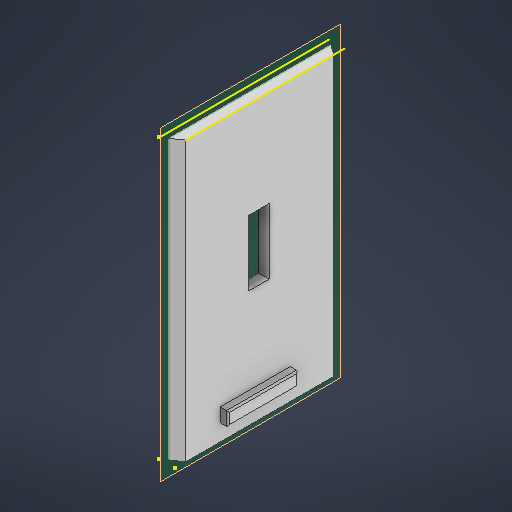
# Autodesk Inventor part: Part2
Saved by Autodesk Inventor 2026.1 (Build 301233000, 233)
## iProperties
Created: 2025-08-25
Part Number: Part2
Material: Generic
Document SubType Name: Modeling
Designer: usman
Density: 1 g/cm^3
Appearance: Default
Author: usman
Autodesk Inventor part; units mm, degrees
(part 1 of 2)
ref_plane "YZ Plane" through (0, 0, 0) normal (1, 0, 0) x (0, 1, 0)
ref_plane "XZ Plane" through (0, 0, 0) normal (0, 1, 0) x (-1, 0, 0)
ref_plane "XY Plane" through (0, 0, 0) normal (0, 0, 1) x (1, 0, 0)
sketch "Sketch1" plane through (0, 0, 0) normal (1, 0, 0) x (0, 1, 0)
  line L0 (0, 0) -> (178.9, 0)
  line L1 (178.9, 0) -> (178.9, -109)
  line L2 (178.9, -109) -> (0, -109)
  line L3 (0, -109) -> (0, 0)
  dimension "d0" = 178.9
  dimension "d1" = 109
  constraints: 8 end point, 2 parallel, 1 horizontal, 1 perpendicular
  measures "d0" distance of L1.end L2.end
  measures "d1" distance of L0.end L1.end
extrude "Extrusion1" add sketch "Sketch1" along normal blind 10
sketch "Sketch2" plane through (0, 178.9, 0) normal (0, 1, 0) x (1, 0, 0)
  point P0 (0, 0)
sketch "Sketch3" plane through (0, 178.9, 0) normal (0, 1, 0) x (1, 0, 0)
  line L0 (0, 109) -> (10, 101.9979)
  line L1 (10, 109) -> (10, 0) projected
  line L2 (0, 109) -> (0, 0) projected
  line L3 (0, 0) -> (10, 0) projected
  line L4 (0, 0) -> (10, 7.0021)
  dimension "d4" = 125
  dimension "d5" = 125
  constraints: 4 end point, 2 point on line
  measures "d4" angle of L2 L0
  measures "d5" angle of L2 L4
extrude "Extrusion2" cut sketch "Sketch3" against normal through all contours L4 L1 L3
sketch "Sketch4" plane through (0, 178.9, -109) normal (0, 1, 0) x (1, 0, 0)
  point P0 (0, -109)
sketch "Sketch5" plane through (0, 178.9, -109) normal (0, 1, 0) x (1, 0, 0)
  line L0 (0, -109) -> (0, 0) projected
  line L1 (10, 0) -> (10, -101.9979) projected
sketch "Sketch6" plane through (0, 178.9, -109) normal (0, 1, 0) x (1, 0, 0)
  line L0 (0, -109) -> (0, 0) projected
  line L1 (0, 0) -> (10, -7.0021)
  line L2 (10, 0) -> (10, -101.9979) projected
  line L3 (0, 0) -> (10, 0)
  line L4 (0, 0) -> (10, 0) projected
  line L5 (10, 0) -> (10, -7.0021)
  dimension "d8" = 125
  constraints: 6 end point, 1 collinear, 1 perpendicular, 1 point on line
  measures "d8" angle of L2 L1
extrude "Extrusion3" cut sketch "Sketch6" against normal through all
sketch "Sketch7" plane through (10, 0, 0) normal (1, 0, 0) x (0, 0, -1)
  point P0 (0, 0)
sketch "Sketch8" plane through (10, 0, 0) normal (1, 0, 0) x (0, 0, -1)
  line L0 (47.4589, 116.9) -> (60.4589, 116.9)
  line L1 (60.4589, 116.9) -> (60.4589, 74.9)
  line L2 (60.4589, 74.9) -> (47.4589, 74.9)
  line L3 (47.4589, 74.9) -> (47.4589, 116.9)
  line L4 (101.9979, 178.9) -> (7.0021, 178.9) projected
  point P0 (0, 0)
  dimension "d11" = 13
  dimension "d12" = 42
  dimension "d13" = 62
  constraints: 8 end point, 2 parallel, 1 horizontal, 1 perpendicular
  measures "d11" distance of L0.start L0.end
  measures "d12" distance of L0.end L1.end
  measures "d13" distance between parallel lines of L0 L4
extrude "Extrusion4" cut sketch "Sketch8" against normal through all
sketch "Sketch9" plane through (0, 0, 0) normal (0.5735764, 0, 0.819152) x (0.819152, 0, -0.5735764)
  point P0 (0, 0)
sketch "Sketch10" plane through (0, 0, 0) normal (0.5735764, 0, 0.819152) x (0.819152, 0, -0.5735764)
  point P0 (0, 0)
sketch "Sketch11" plane through (0, 178.9, 0) normal (0, 1, 0) x (1, 0, 0)
  line L0 (0, 109) -> (0, 0) projected
  line L1 (0, 109) -> (0.5, 109)
  line L2 (0.5, 109) -> (0.5, 0)
  line L3 (0.5, 0) -> (0, 0)
  line L4 (0, 0) -> (0, 109)
  dimension "d16" = 0.5
  constraints: 8 end point, 2 parallel, 1 horizontal, 1 perpendicular
  measures "d16" distance of L2.end L3.end
extrude "Extrusion5" cut sketch "Sketch11" against normal through all
sketch "Sketch12" plane through (10, 0, 0) normal (1, 0, 0) x (0, 0, -1)
  line L0 (73.9981, 10.7247) -> (29.0021, 10.7247)
  line L1 (29.0021, 10.7247) -> (29.0021, 19.4458)
  line L2 (29.0021, 19.4458) -> (73.9981, 19.4458)
  line L3 (73.9981, 19.4458) -> (73.9981, 10.7247)
  line L4 (7.0021, 178.9) -> (7.0021, 0) projected
  point P0 (0, 0)
  point P1 (29.0021, 15.0853)
  dimension "d19" = 22
  dimension "d20" = 44.996
  constraints: 8 end point, 2 parallel, 1 horizontal, 1 midpoint, 1 perpendicular
  measures "d19" distance from line of L4 point (29.002, 15.085)
  measures "d20" distance of L0.start L0.end
extrude "Extrusion6" add sketch "Sketch12" along normal blind 5
fillet "Fillet1" radius 1 4 edges at (15, 19.4458, -51.5001) (15, 10.7247, -51.5001) (15, 15.0853, -29.0021) (15, 15.0853, -73.9981)
sketch "Sketch14" plane through (10, 178.9, -7.0021) normal (0, 1, 0) x (1, 0, 0)
  line L0 (0, 94.9958) -> (-9.5, 101.6478) projected
  line L1 (-9.5, 101.6478) -> (-7, 101.6478)
  line L2 (-7, 101.6478) -> (-7, -6.652)
  line L3 (-7, -6.652) -> (-9.5, -6.652)
  line L4 (-9.5, -6.652) -> (-9.5, 101.6478)
  point P0 (-10, -7.0021)
  dimension "d25" = 2.5
  constraints: 8 end point, 2 parallel, 1 horizontal, 1 perpendicular
  measures "d25" distance of L2.end L3.end
extrude "Extrusion7" cut sketch "Sketch14" against normal through all
ref_plane "Work Plane2" through (4, 178.9, -106.8994) normal (-1, 0, 0) x (0, 0, 1)
sketch "Sketch15" plane through (4, 178.9, -106.8994) normal (-1, 0, 0) x (0, 0, 1)
  arc A0 (103.1758, -166.633) -> (98.1758, -166.633) centre (100.6758, -166.633) ccw
  arc A1 (6.623, -166.633) -> (1.623, -166.633) centre (4.123, -166.633) ccw
  line L0 (104.7988, -178.9) -> (0, -178.9) projected
  line L1 (104.7988, 0) -> (104.7988, -178.9) projected
  line L2 (0, -178.9) -> (0, 0) projected
  line L3 (103.1758, -166.633) -> (98.1758, -166.633)
  line L4 (6.623, -166.633) -> (1.623, -166.633)
  point P0 (106.8994, -178.9)
  dimension "d29" = 12.267
  dimension "d30" = 12.267
  dimension "d31" = 4.123
  dimension "d32" = 4.123
  dimension "d33" = 5
  dimension "d34" = 5
  constraints: 4 end point, 4 point on circle, 2 centre point, 2 point on line, 1 horizontal
  measures "d29" distance from line of A0.centre L0
  measures "d30" distance from line of A1.centre L0
  measures "d31" distance from line of A0.centre L1
  measures "d32" distance from line of L2 A1.centre
  measures "d33" diameter of A0
  measures "d34" diameter of A1
revolve "Revolution1" add sketch "Sketch15" angle 360 about axis through (4, 12.267, -3.7236) along (0, 0, -1)
sketch "Sketch18" plane through (3, 178.9, -106.8994) normal (-1, 0, 0) x (0, 0, 1)
  line L0 (10.7042, -119.5303) -> (95.1976, -119.5303) construction
  line L1 (95.1976, -119.5303) -> (95.1976, -169.3697) construction
  line L2 (95.1976, -169.3697) -> (10.7042, -169.3697) construction
  line L3 (10.7042, -169.3697) -> (10.7042, -119.5303) construction
  line L4 (38.2413, -134.9776) -> (35.8706, -134.9776)
  line L5 (35.8706, -134.9776) -> (35.4573, -135.9339)
  spline S0 degree 2 poles (35.4573, -135.9339) (35.3029, -136.2925) (35.3029, -136.4668) knots 0 0 0 1 1 1
  spline S1 degree 2 poles (35.3029, -136.4668) (35.3029, -136.6062) (35.5718, -136.8204) (36.0101, -136.8503) knots 0 0 0 1 2 2 2
  line L6 (36.0101, -136.8503) -> (36.0101, -137.0146)
  line L7 (36.0101, -137.0146) -> (34.0877, -137.0146)
  line L8 (34.0877, -137.0146) -> (34.0877, -136.8503)
  spline S2 degree 2 poles (34.0877, -136.8503) (34.4711, -136.7805) (34.5807, -136.6759) knots 0 0 0 1 1 1
  spline S3 degree 2 poles (34.5807, -136.6759) (34.8098, -136.4568) (35.0887, -135.7944) knots 0 0 0 1 1 1
  line L9 (35.0887, -135.7944) -> (37.2402, -130.7792)
  line L10 (37.2402, -130.7792) -> (37.3996, -130.7792)
  line L11 (37.3996, -130.7792) -> (39.5213, -135.8492)
  spline S4 degree 2 poles (39.5213, -135.8492) (39.7753, -136.4618) (40.1936, -136.8254) (40.5671, -136.8503) knots 0 0 0 1 2 2 2
  line L12 (40.5671, -136.8503) -> (40.5671, -137.0146)
  line L13 (40.5671, -137.0146) -> (38.1616, -137.0146)
  line L14 (38.1616, -137.0146) -> (38.1616, -136.8503)
  spline S5 degree 2 poles (38.1616, -136.8503) (38.5252, -136.8303) (38.7842, -136.6261) (38.7842, -136.4767) knots 0 0 0 1 2 2 2
  spline S6 degree 2 poles (38.7842, -136.4767) (38.7842, -136.2775) (38.6049, -135.8492) knots 0 0 0 1 1 1
  line L15 (38.6049, -135.8492) -> (38.2413, -134.9776)
  line L16 (38.1019, -134.6439) -> (37.0759, -132.1786)
  line L17 (37.0759, -132.1786) -> (36.0101, -134.6439)
  line L18 (36.0101, -134.6439) -> (38.1019, -134.6439)
  line L19 (44.666, -130.9186) -> (44.3174, -131.6806)
  line L20 (44.3174, -131.6806) -> (42.4846, -131.6806)
  line L21 (42.4846, -131.6806) -> (42.0812, -132.4974)
  spline S7 degree 2 poles (42.0812, -132.4974) (43.2715, -132.6717) (43.9688, -133.3839) knots 0 0 0 1 1 1
  spline S8 degree 2 poles (43.9688, -133.3839) (44.5664, -133.9965) (44.5664, -134.8232) knots 0 0 0 1 1 1
  spline S9 degree 2 poles (44.5664, -134.8232) (44.5664, -135.3014) (44.173, -136.1231) (43.5803, -136.6959) (43.2167, -136.8702) knots 0 0 0 1 2 3 3 3
  spline S10 degree 2 poles (43.2167, -136.8702) (42.6988, -137.1192) (42.1559, -137.1192) knots 0 0 0 1 1 1
  spline S11 degree 2 poles (42.1559, -137.1192) (41.6031, -137.1192) (41.105, -136.7457) (41.105, -136.5216) knots 0 0 0 1 2 2 2
  spline S12 degree 2 poles (41.105, -136.5216) (41.105, -136.397) (41.3092, -136.2028) (41.4686, -136.2028) knots 0 0 0 1 2 2 2
  spline S13 degree 2 poles (41.4686, -136.2028) (41.5831, -136.2028) (41.7624, -136.2775) (41.9716, -136.4269) knots 0 0 0 1 2 2 2
  spline S14 degree 2 poles (41.9716, -136.4269) (42.3103, -136.656) (42.6589, -136.661) knots 0 0 0 1 1 1
  spline S15 degree 2 poles (42.6589, -136.661) (43.1819, -136.661) (43.9837, -135.8641) (43.9837, -135.2914) knots 0 0 0 1 2 2 2
  spline S16 degree 2 poles (43.9837, -135.2914) (43.9837, -134.7386) (43.2715, -133.7774) (42.644, -133.5184) knots 0 0 0 1 2 2 2
  spline S17 degree 2 poles (42.644, -133.5184) (42.1559, -133.3142) (41.3092, -133.2843) knots 0 0 0 1 1 1
  line L22 (41.3092, -133.2843) -> (42.4796, -130.9186)
  line L23 (42.4796, -130.9186) -> (44.666, -130.9186)
  spline S18 degree 2 poles (45.6073, -134.0015) (45.6073, -132.9606) (46.2348, -131.4565) (46.7578, -131.0879) knots 0 0 0 1 2 2 2
  spline S19 degree 2 poles (46.7578, -131.0879) (47.1612, -130.7941) (47.5945, -130.7941) knots 0 0 0 1 1 1
  spline S20 degree 2 poles (47.5945, -130.7941) (48.2967, -130.7941) (48.8545, -131.5063) knots 0 0 0 1 1 1
  spline S21 degree 2 poles (48.8545, -131.5063) (49.5518, -132.3928) (49.5518, -133.9068) knots 0 0 0 1 1 1
  spline S22 degree 2 poles (49.5518, -133.9068) (49.5518, -134.9677) (48.9392, -136.4518) (47.9929, -137.1192) (47.5497, -137.1192) knots 0 0 0 1 2 3 3 3
  spline S23 degree 2 poles (47.5497, -137.1192) (46.6781, -137.1192) (46.0954, -136.0883) knots 0 0 0 1 1 1
  spline S24 degree 2 poles (46.0954, -136.0883) (45.6073, -135.2217) (45.6073, -134.0015) knots 0 0 0 1 1 1
  spline S25 degree 2 poles (46.4888, -134.116) (46.4888, -135.3711) (46.7976, -136.1679) knots 0 0 0 1 1 1
  spline S26 degree 2 poles (46.7976, -136.1679) (47.0566, -136.8353) (47.5646, -136.8353) knots 0 0 0 1 1 1
  spline S27 degree 2 poles (47.5646, -136.8353) (47.8086, -136.8353) (48.3266, -136.402) (48.4611, -135.889) knots 0 0 0 1 2 2 2
  spline S28 degree 2 poles (48.4611, -135.889) (48.6702, -135.1171) (48.6702, -133.7126) knots 0 0 0 1 1 1
  spline S29 degree 2 poles (48.6702, -133.7126) (48.6702, -132.6667) (48.4561, -131.9745) knots 0 0 0 1 1 1
  spline S30 degree 2 poles (48.4561, -131.9745) (48.2917, -131.4565) (48.0377, -131.2423) knots 0 0 0 1 1 1
  spline S31 degree 2 poles (48.0377, -131.2423) (47.8535, -131.0929) (47.5895, -131.0929) knots 0 0 0 1 1 1
  spline S32 degree 2 poles (47.5895, -131.0929) (47.2857, -131.0929) (47.0466, -131.3668) knots 0 0 0 1 1 1
  spline S33 degree 2 poles (47.0466, -131.3668) (46.7229, -131.7404) (46.4888, -133.3391) (46.4888, -134.116) knots 0 0 0 1 2 2 2
  spline S34 degree 2 poles (50.2142, -134.0015) (50.2142, -132.9606) (50.8417, -131.4565) (51.3646, -131.0879) knots 0 0 0 1 2 2 2
  spline S35 degree 2 poles (51.3646, -131.0879) (51.7681, -130.7941) (52.2013, -130.7941) knots 0 0 0 1 1 1
  spline S36 degree 2 poles (52.2013, -130.7941) (52.9036, -130.7941) (53.4614, -131.5063) knots 0 0 0 1 1 1
  spline S37 degree 2 poles (53.4614, -131.5063) (54.1586, -132.3928) (54.1586, -133.9068) knots 0 0 0 1 1 1
  spline S38 degree 2 poles (54.1586, -133.9068) (54.1586, -134.9677) (53.5461, -136.4518) (52.5998, -137.1192) (52.1565, -137.1192) knots 0 0 0 1 2 3 3 3
  spline S39 degree 2 poles (52.1565, -137.1192) (51.285, -137.1192) (50.7022, -136.0883) knots 0 0 0 1 1 1
  spline S40 degree 2 poles (50.7022, -136.0883) (50.2142, -135.2217) (50.2142, -134.0015) knots 0 0 0 1 1 1
  spline S41 degree 2 poles (51.0957, -134.116) (51.0957, -135.3711) (51.4045, -136.1679) knots 0 0 0 1 1 1
  spline S42 degree 2 poles (51.4045, -136.1679) (51.6635, -136.8353) (52.1715, -136.8353) knots 0 0 0 1 1 1
  spline S43 degree 2 poles (52.1715, -136.8353) (52.4155, -136.8353) (52.9335, -136.402) (53.0679, -135.889) knots 0 0 0 1 2 2 2
  spline S44 degree 2 poles (53.0679, -135.889) (53.2771, -135.1171) (53.2771, -133.7126) knots 0 0 0 1 1 1
  spline S45 degree 2 poles (53.2771, -133.7126) (53.2771, -132.6667) (53.063, -131.9745) knots 0 0 0 1 1 1
  spline S46 degree 2 poles (53.063, -131.9745) (52.8986, -131.4565) (52.6446, -131.2423) knots 0 0 0 1 1 1
  spline S47 degree 2 poles (52.6446, -131.2423) (52.4603, -131.0929) (52.1964, -131.0929) knots 0 0 0 1 1 1
  spline S48 degree 2 poles (52.1964, -131.0929) (51.8926, -131.0929) (51.6535, -131.3668) knots 0 0 0 1 1 1
  spline S49 degree 2 poles (51.6535, -131.3668) (51.3298, -131.7404) (51.0957, -133.3391) (51.0957, -134.116) knots 0 0 0 1 2 2 2
  line L24 (59.1739, -138.9968) -> (54.4126, -138.9968)
  line L25 (54.4126, -138.9968) -> (54.4126, -138.6183)
  line L26 (54.4126, -138.6183) -> (59.1739, -138.6183)
  line L27 (59.1739, -138.6183) -> (59.1739, -138.9968)
  line L28 (64.3734, -135.3263) -> (64.5228, -135.3561)
  line L29 (64.5228, -135.3561) -> (63.9999, -137.0146)
  line L30 (63.9999, -137.0146) -> (59.2835, -137.0146)
  line L31 (59.2835, -137.0146) -> (59.2835, -136.8503)
  line L32 (59.2835, -136.8503) -> (59.5126, -136.8503)
  spline S50 degree 2 poles (59.5126, -136.8503) (59.8961, -136.8503) (60.0604, -136.5963) knots 0 0 0 1 1 1
  spline S51 degree 2 poles (60.0604, -136.5963) (60.155, -136.4568) (60.155, -135.9339) knots 0 0 0 1 1 1
  line L33 (60.155, -135.9339) -> (60.155, -131.9994)
  spline S52 degree 2 poles (60.155, -131.9994) (60.155, -131.4266) (60.0305, -131.2822) knots 0 0 0 1 1 1
  spline S53 degree 2 poles (60.0305, -131.2822) (59.8562, -131.083) (59.5126, -131.083) knots 0 0 0 1 1 1
  line L34 (59.5126, -131.083) -> (59.2835, -131.083)
  line L35 (59.2835, -131.083) -> (59.2835, -130.9186)
  line L36 (59.2835, -130.9186) -> (62.0376, -130.9186)
  line L37 (62.0376, -130.9186) -> (62.0376, -131.083)
  spline S54 degree 2 poles (62.0376, -131.083) (61.5495, -131.078) (61.1611, -131.2672) (61.0166, -131.5561) (61.0166, -132.099) knots 0 0 0 1 2 3 3 3
  line L38 (61.0166, -132.099) -> (61.0166, -135.9289)
  spline S55 degree 2 poles (61.0166, -135.9289) (61.0166, -136.3024) (61.0864, -136.4419) knots 0 0 0 1 1 1
  spline S56 degree 2 poles (61.0864, -136.4419) (61.1411, -136.5365) (61.3653, -136.6261) (61.9579, -136.6261) knots 0 0 0 1 2 2 2
  line L39 (61.9579, -136.6261) -> (62.4012, -136.6261)
  spline S57 degree 2 poles (62.4012, -136.6261) (63.1034, -136.6261) (63.6712, -136.417) (64.1393, -135.894) (64.3734, -135.3263) knots 0 0 0 1 2 3 3 3
  line L40 (66.4253, -132.7763) -> (66.4253, -136.0833)
  spline S58 degree 2 poles (66.4253, -136.0833) (66.4253, -136.4668) (66.5349, -136.7257) (66.759, -136.8503) (67.0479, -136.8503) knots 0 0 0 1 2 3 3 3
  line L41 (67.0479, -136.8503) -> (67.0479, -137.0146)
  line L42 (67.0479, -137.0146) -> (65.0508, -137.0146)
  line L43 (65.0508, -137.0146) -> (65.0508, -136.8503)
  spline S59 degree 2 poles (65.0508, -136.8503) (65.3496, -136.8503) (65.5588, -136.7357) (65.6783, -136.4668) (65.6783, -136.0833) knots 0 0 0 1 2 3 3 3
  line L44 (65.6783, -136.0833) -> (65.6783, -134.4995)
  spline S60 degree 2 poles (65.6783, -134.4995) (65.6783, -133.8321) (65.6384, -133.6329) knots 0 0 0 1 1 1
  spline S61 degree 2 poles (65.6384, -133.6329) (65.6086, -133.4885) (65.4691, -133.3739) (65.3546, -133.3739) knots 0 0 0 1 2 2 2
  spline S62 degree 2 poles (65.3546, -133.3739) (65.2301, -133.3739) (65.0508, -133.4437) knots 0 0 0 1 1 1
  line L45 (65.0508, -133.4437) -> (64.986, -133.2793)
  line L46 (64.986, -133.2793) -> (66.2261, -132.7763)
  line L47 (66.2261, -132.7763) -> (66.4253, -132.7763)
  spline S63 degree 2 poles (66.0518, -130.6198) (66.2411, -130.6198) (66.505, -130.8837) (66.505, -131.073) knots 0 0 0 1 2 2 2
  spline S64 degree 2 poles (66.505, -131.073) (66.505, -131.2623) (66.2411, -131.5312) (66.0518, -131.5312) knots 0 0 0 1 2 2 2
  spline S65 degree 2 poles (66.0518, -131.5312) (65.8626, -131.5312) (65.5936, -131.2623) (65.5936, -131.073) knots 0 0 0 1 2 2 2
  spline S66 degree 2 poles (65.5936, -131.073) (65.5936, -130.8837) (65.8576, -130.6198) (66.0518, -130.6198) knots 0 0 0 1 2 2 2
  spline S67 degree 2 poles (70.4694, -136.5514) (70.1706, -136.8652) (69.5929, -137.1391) (69.2592, -137.1391) knots 0 0 0 1 2 2 2
  spline S68 degree 2 poles (69.2592, -137.1391) (68.5868, -137.1391) (67.5808, -136.0136) (67.5808, -135.127) knots 0 0 0 1 2 2 2
  spline S69 degree 2 poles (67.5808, -135.127) (67.5808, -134.2455) (68.6964, -132.7763) (69.573, -132.7763) knots 0 0 0 1 2 2 2
  spline S70 degree 2 poles (69.573, -132.7763) (70.1158, -132.7763) (70.4694, -133.1249) knots 0 0 0 1 1 1
  line L48 (70.4694, -133.1249) -> (70.4694, -132.353)
  spline S71 degree 2 poles (70.4694, -132.353) (70.4694, -131.6507) (70.3997, -131.332) (70.2602, -131.2174) (70.1507, -131.2174) knots 0 0 0 1 2 3 3 3
  spline S72 degree 2 poles (70.1507, -131.2174) (70.0361, -131.2174) (69.8419, -131.2872) knots 0 0 0 1 1 1
  line L49 (69.8419, -131.2872) -> (69.7821, -131.1228)
  line L50 (69.7821, -131.1228) -> (71.0073, -130.6198)
  line L51 (71.0073, -130.6198) -> (71.2115, -130.6198)
  line L52 (71.2115, -130.6198) -> (71.2115, -135.386)
  spline S73 degree 2 poles (71.2115, -135.386) (71.2115, -136.1032) (71.2812, -136.4219) (71.4257, -136.5465) (71.5253, -136.5465) knots 0 0 0 1 2 3 3 3
  spline S74 degree 2 poles (71.5253, -136.5465) (71.6448, -136.5465) (71.849, -136.4717) knots 0 0 0 1 1 1
  line L53 (71.849, -136.4717) -> (71.8988, -136.6361)
  line L54 (71.8988, -136.6361) -> (70.6786, -137.1391)
  line L55 (70.6786, -137.1391) -> (70.4694, -137.1391)
  line L56 (70.4694, -137.1391) -> (70.4694, -136.5514)
  line L57 (70.4694, -136.2327) -> (70.4694, -134.121)
  spline S75 degree 2 poles (70.4694, -134.121) (70.4445, -133.8122) (70.1706, -133.3092) (69.7273, -133.0552) (69.5182, -133.0552) knots 0 0 0 1 2 3 3 3
  spline S76 degree 2 poles (69.5182, -133.0552) (69.1197, -133.0552) (68.811, -133.4088) knots 0 0 0 1 1 1
  spline S77 degree 2 poles (68.811, -133.4088) (68.4026, -133.877) (68.4026, -134.7734) knots 0 0 0 1 1 1
  spline S78 degree 2 poles (68.4026, -134.7734) (68.4026, -135.6799) (69.1944, -136.6461) (69.6775, -136.6461) knots 0 0 0 1 2 2 2
  spline S79 degree 2 poles (69.6775, -136.6461) (70.0859, -136.6461) (70.4694, -136.2327) knots 0 0 0 1 1 1
  line L58 (17.7843, -140.4209) -> (17.7843, -142.5276)
  line L59 (17.7843, -142.5276) -> (17.62, -142.5276)
  spline S80 degree 2 poles (17.62, -142.5276) (17.5403, -141.9199) (17.117, -141.2028) (16.345, -140.7794) (15.9267, -140.7794) knots 0 0 0 1 2 3 3 3
  spline S81 degree 2 poles (15.9267, -140.7794) (15.4585, -140.7794) (14.8459, -141.3522) (14.8459, -141.7158) knots 0 0 0 1 2 2 2
  spline S82 degree 2 poles (14.8459, -141.7158) (14.8459, -141.9947) (15.0401, -142.2238) knots 0 0 0 1 1 1
  spline S83 degree 2 poles (15.0401, -142.2238) (15.319, -142.5624) (16.3699, -143.1252) knots 0 0 0 1 1 1
  spline S84 degree 2 poles (16.3699, -143.1252) (17.2216, -143.5834) (17.8491, -144.0715) (18.1878, -144.7389) (18.1878, -145.1024) knots 0 0 0 1 2 3 3 3
  spline S85 degree 2 poles (18.1878, -145.1024) (18.1878, -145.7947) (17.112, -146.7958) (16.2653, -146.7958) knots 0 0 0 1 2 2 2
  spline S86 degree 2 poles (16.2653, -146.7958) (16.0014, -146.7958) (15.7673, -146.7559) knots 0 0 0 1 1 1
  spline S87 degree 2 poles (15.7673, -146.7559) (15.6278, -146.731) (14.7513, -146.4471) (14.6318, -146.4471) knots 0 0 0 1 2 2 2
  spline S88 degree 2 poles (14.6318, -146.4471) (14.5222, -146.4471) (14.3877, -146.5816) (14.3578, -146.7958) knots 0 0 0 1 2 2 2
  line L60 (14.3578, -146.7958) -> (14.1935, -146.7958)
  line L61 (14.1935, -146.7958) -> (14.1935, -144.704)
  line L62 (14.1935, -144.704) -> (14.3578, -144.704)
  spline S89 degree 2 poles (14.3578, -144.704) (14.4724, -145.3614) (14.8708, -146.0138) (15.6876, -146.4471) (16.1707, -146.4471) knots 0 0 0 1 2 3 3 3
  spline S90 degree 2 poles (16.1707, -146.4471) (16.7335, -146.4471) (17.3859, -145.8545) (17.3859, -145.4461) knots 0 0 0 1 2 2 2
  spline S91 degree 2 poles (17.3859, -145.4461) (17.3859, -145.2219) (17.1369, -144.7638) (16.8779, -144.5645) knots 0 0 0 1 2 2 2
  spline S92 degree 2 poles (16.8779, -144.5645) (16.7036, -144.4301) (15.1348, -143.5535) (14.4724, -143.0306) (14.1287, -142.403) (14.1287, -142.0245) knots 0 0 0 1 2 3 4 4 4
  spline S93 degree 2 poles (14.1287, -142.0245) (14.1287, -141.3671) (15.1398, -140.4209) (15.9217, -140.4209) knots 0 0 0 1 2 2 2
  spline S94 degree 2 poles (15.9217, -140.4209) (16.4048, -140.4209) (16.9526, -140.6599) knots 0 0 0 1 1 1
  spline S95 degree 2 poles (16.9526, -140.6599) (17.2066, -140.7695) (17.3112, -140.7695) knots 0 0 0 1 1 1
  spline S96 degree 2 poles (17.3112, -140.7695) (17.4258, -140.7695) (17.5752, -140.63) (17.62, -140.4209) knots 0 0 0 1 2 2 2
  line L63 (17.62, -140.4209) -> (17.7843, -140.4209)
  spline S97 degree 2 poles (19.652, -144.0914) (19.647, -145.0078) (20.0952, -145.5258) knots 0 0 0 1 1 1
  spline S98 degree 2 poles (20.0952, -145.5258) (20.5485, -146.0487) (21.1561, -146.0487) knots 0 0 0 1 1 1
  spline S99 degree 2 poles (21.1561, -146.0487) (21.5595, -146.0487) (22.1571, -145.6054) (22.3613, -145.0626) knots 0 0 0 1 2 2 2
  line L64 (22.3613, -145.0626) -> (22.5008, -145.1522)
  spline S100 degree 2 poles (22.5008, -145.1522) (22.4061, -145.7698) (21.4997, -146.7808) (20.8124, -146.7808) knots 0 0 0 1 2 2 2
  spline S101 degree 2 poles (20.8124, -146.7808) (20.0703, -146.7808) (19.0145, -145.6254) (19.0145, -144.6542) knots 0 0 0 1 2 2 2
  spline S102 degree 2 poles (19.0145, -144.6542) (19.0145, -143.5983) (20.1002, -142.418) (20.917, -142.418) knots 0 0 0 1 2 2 2
  spline S103 degree 2 poles (20.917, -142.418) (21.6093, -142.418) (22.5008, -143.3294) (22.5008, -144.0914) knots 0 0 0 1 2 2 2
  line L65 (22.5008, -144.0914) -> (19.652, -144.0914)
  line L66 (19.652, -143.8324) -> (21.5645, -143.8324)
  spline S104 degree 2 poles (21.5645, -143.8324) (21.5396, -143.439) (21.4698, -143.2746) knots 0 0 0 1 1 1
  spline S105 degree 2 poles (21.4698, -143.2746) (21.3553, -143.0256) (20.912, -142.7367) (20.668, -142.7367) knots 0 0 0 1 2 2 2
  spline S106 degree 2 poles (20.668, -142.7367) (20.2945, -142.7367) (19.7018, -143.3145) (19.652, -143.8324) knots 0 0 0 1 2 2 2
  line L67 (24.2589, -142.418) -> (24.2589, -143.3443)
  spline S107 degree 2 poles (24.2589, -143.3443) (24.7768, -142.418) (25.3197, -142.418) knots 0 0 0 1 1 1
  spline S108 degree 2 poles (25.3197, -142.418) (25.5637, -142.418) (25.8874, -142.7168) (25.8874, -142.916) knots 0 0 0 1 2 2 2
  spline S109 degree 2 poles (25.8874, -142.916) (25.8874, -143.0903) (25.6534, -143.3344) (25.494, -143.3344) knots 0 0 0 1 2 2 2
  spline S110 degree 2 poles (25.494, -143.3344) (25.3346, -143.3344) (24.9461, -143.0256) (24.8515, -143.0256) knots 0 0 0 1 2 2 2
  spline S111 degree 2 poles (24.8515, -143.0256) (24.7718, -143.0256) (24.6772, -143.1152) knots 0 0 0 1 1 1
  spline S112 degree 2 poles (24.6772, -143.1152) (24.473, -143.2995) (24.2589, -143.7229) knots 0 0 0 1 1 1
  line L68 (24.2589, -143.7229) -> (24.2589, -145.6951)
  spline S113 degree 2 poles (24.2589, -145.6951) (24.2589, -146.0387) (24.3435, -146.213) knots 0 0 0 1 1 1
  spline S114 degree 2 poles (24.3435, -146.213) (24.4033, -146.3326) (24.6971, -146.4919) (24.976, -146.4919) knots 0 0 0 1 2 2 2
  line L69 (24.976, -146.4919) -> (24.976, -146.6563)
  line L70 (24.976, -146.6563) -> (22.8643, -146.6563)
  line L71 (22.8643, -146.6563) -> (22.8643, -146.4919)
  spline S115 degree 2 poles (22.8643, -146.4919) (23.1781, -146.4919) (23.3325, -146.3923) knots 0 0 0 1 1 1
  spline S116 degree 2 poles (23.3325, -146.3923) (23.4421, -146.3226) (23.4869, -146.1632) knots 0 0 0 1 1 1
  spline S117 degree 2 poles (23.4869, -146.1632) (23.5118, -146.0836) (23.5118, -145.725) knots 0 0 0 1 1 1
  line L72 (23.5118, -145.725) -> (23.5118, -144.1362)
  spline S118 degree 2 poles (23.5118, -144.1362) (23.5118, -143.419) (23.452, -143.1451) (23.2976, -143.0156) (23.1781, -143.0156) knots 0 0 0 1 2 3 3 3
  spline S119 degree 2 poles (23.1781, -143.0156) (23.0387, -143.0156) (22.8643, -143.0854) knots 0 0 0 1 1 1
  line L73 (22.8643, -143.0854) -> (22.8195, -142.921)
  line L74 (22.8195, -142.921) -> (24.0696, -142.418)
  line L75 (24.0696, -142.418) -> (24.2589, -142.418)
  line L76 (27.536, -142.418) -> (27.536, -145.725)
  spline S120 degree 2 poles (27.536, -145.725) (27.536, -146.1085) (27.6455, -146.3674) (27.8696, -146.4919) (28.1585, -146.4919) knots 0 0 0 1 2 3 3 3
  line L77 (28.1585, -146.4919) -> (28.1585, -146.6563)
  line L78 (28.1585, -146.6563) -> (26.1614, -146.6563)
  line L79 (26.1614, -146.6563) -> (26.1614, -146.4919)
  spline S121 degree 2 poles (26.1614, -146.4919) (26.4602, -146.4919) (26.6694, -146.3774) (26.7889, -146.1085) (26.7889, -145.725) knots 0 0 0 1 2 3 3 3
  line L80 (26.7889, -145.725) -> (26.7889, -144.1412)
  spline S122 degree 2 poles (26.7889, -144.1412) (26.7889, -143.4738) (26.749, -143.2746) knots 0 0 0 1 1 1
  spline S123 degree 2 poles (26.749, -143.2746) (26.7192, -143.1302) (26.5797, -143.0156) (26.4652, -143.0156) knots 0 0 0 1 2 2 2
  spline S124 degree 2 poles (26.4652, -143.0156) (26.3407, -143.0156) (26.1614, -143.0854) knots 0 0 0 1 1 1
  line L81 (26.1614, -143.0854) -> (26.0966, -142.921)
  line L82 (26.0966, -142.921) -> (27.3367, -142.418)
  line L83 (27.3367, -142.418) -> (27.536, -142.418)
  spline S125 degree 2 poles (27.1624, -140.2615) (27.3517, -140.2615) (27.6156, -140.5254) (27.6156, -140.7147) knots 0 0 0 1 2 2 2
  spline S126 degree 2 poles (27.6156, -140.7147) (27.6156, -140.9039) (27.3517, -141.1729) (27.1624, -141.1729) knots 0 0 0 1 2 2 2
  spline S127 degree 2 poles (27.1624, -141.1729) (26.9732, -141.1729) (26.7042, -140.9039) (26.7042, -140.7147) knots 0 0 0 1 2 2 2
  spline S128 degree 2 poles (26.7042, -140.7147) (26.7042, -140.5254) (26.9682, -140.2615) (27.1624, -140.2615) knots 0 0 0 1 2 2 2
  spline S129 degree 2 poles (31.0073, -146.0587) (30.3748, -146.5517) (30.2104, -146.6264) knots 0 0 0 1 1 1
  spline S130 degree 2 poles (30.2104, -146.6264) (29.9714, -146.741) (29.6974, -146.741) knots 0 0 0 1 1 1
  spline S131 degree 2 poles (29.6974, -146.741) (29.2691, -146.741) (28.7163, -146.1583) (28.7163, -145.6801) knots 0 0 0 1 2 2 2
  spline S132 degree 2 poles (28.7163, -145.6801) (28.7163, -145.3813) (28.8508, -145.1572) knots 0 0 0 1 1 1
  spline S133 degree 2 poles (28.8508, -145.1572) (29.035, -144.8534) (29.9465, -144.3155) (31.0073, -143.927) knots 0 0 0 1 2 2 2
  line L84 (31.0073, -143.927) -> (31.0073, -143.7677)
  spline S134 degree 2 poles (31.0073, -143.7677) (31.0073, -143.1501) (30.6188, -142.6919) (30.2453, -142.6919) knots 0 0 0 1 2 2 2
  spline S135 degree 2 poles (30.2453, -142.6919) (29.9664, -142.6919) (29.797, -142.8463) knots 0 0 0 1 1 1
  spline S136 degree 2 poles (29.797, -142.8463) (29.6277, -142.9957) (29.6277, -143.1949) knots 0 0 0 1 1 1
  line L85 (29.6277, -143.1949) -> (29.6377, -143.4539)
  spline S137 degree 2 poles (29.6377, -143.4539) (29.6377, -143.6631) (29.4235, -143.8872) (29.2542, -143.8872) knots 0 0 0 1 2 2 2
  spline S138 degree 2 poles (29.2542, -143.8872) (29.0898, -143.8872) (28.8757, -143.6531) (28.8757, -143.4489) knots 0 0 0 1 2 2 2
  spline S139 degree 2 poles (28.8757, -143.4489) (28.8757, -143.0654) (29.6676, -142.418) (30.3798, -142.418) knots 0 0 0 1 2 2 2
  spline S140 degree 2 poles (30.3798, -142.418) (30.9276, -142.418) (31.2762, -142.6023) knots 0 0 0 1 1 1
  spline S141 degree 2 poles (31.2762, -142.6023) (31.5452, -142.7417) (31.6697, -143.0356) knots 0 0 0 1 1 1
  spline S142 degree 2 poles (31.6697, -143.0356) (31.7494, -143.2298) (31.7494, -143.8274) knots 0 0 0 1 1 1
  line L86 (31.7494, -143.8274) -> (31.7494, -145.2269)
  spline S143 degree 2 poles (31.7494, -145.2269) (31.7494, -145.8146) (31.7942, -146.0786) (31.8988, -146.1682) (31.9635, -146.1682) knots 0 0 0 1 2 3 3 3
  spline S144 degree 2 poles (31.9635, -146.1682) (32.0382, -146.1682) (32.093, -146.1383) knots 0 0 0 1 1 1
  spline S145 degree 2 poles (32.093, -146.1383) (32.1876, -146.0786) (32.4566, -145.8096) knots 0 0 0 1 1 1
  line L87 (32.4566, -145.8096) -> (32.4566, -146.0587)
  spline S146 degree 2 poles (32.4566, -146.0587) (31.9536, -146.736) (31.4954, -146.736) knots 0 0 0 1 1 1
  spline S147 degree 2 poles (31.4954, -146.736) (31.2712, -146.736) (31.0123, -146.4322) (31.0073, -146.0587) knots 0 0 0 1 2 2 2
  line L88 (31.0073, -145.7698) -> (31.0073, -144.201)
  spline S148 degree 2 poles (31.0073, -144.201) (30.33, -144.4699) (30.1307, -144.5845) knots 0 0 0 1 1 1
  spline S149 degree 2 poles (30.1307, -144.5845) (29.7771, -144.7787) (29.4733, -145.212) (29.4733, -145.466) knots 0 0 0 1 2 2 2
  spline S150 degree 2 poles (29.4733, -145.466) (29.4733, -145.7897) (29.8568, -146.218) (30.1108, -146.218) knots 0 0 0 1 2 2 2
  spline S151 degree 2 poles (30.1108, -146.218) (30.4495, -146.218) (31.0073, -145.7698) knots 0 0 0 1 1 1
  line L89 (34.1848, -140.2615) -> (34.1848, -145.725)
  spline S152 degree 2 poles (34.1848, -145.725) (34.1848, -146.1085) (34.2993, -146.3625) (34.5334, -146.4919) (34.8521, -146.4919) knots 0 0 0 1 2 3 3 3
  line L90 (34.8521, -146.4919) -> (34.8521, -146.6563)
  line L91 (34.8521, -146.6563) -> (32.8251, -146.6563)
  line L92 (32.8251, -146.6563) -> (32.8251, -146.4919)
  spline S153 degree 2 poles (32.8251, -146.4919) (33.109, -146.4919) (33.3182, -146.3774) (33.4377, -146.1085) (33.4377, -145.725) knots 0 0 0 1 2 3 3 3
  line L93 (33.4377, -145.725) -> (33.4377, -141.9847)
  spline S154 degree 2 poles (33.4377, -141.9847) (33.4377, -141.2924) (33.373, -140.9737) (33.2335, -140.8591) (33.1289, -140.8591) knots 0 0 0 1 2 3 3 3
  spline S155 degree 2 poles (33.1289, -140.8591) (33.0094, -140.8591) (32.8301, -140.9289) knots 0 0 0 1 1 1
  line L94 (32.8301, -140.9289) -> (32.7554, -140.7645)
  line L95 (32.7554, -140.7645) -> (33.9806, -140.2615)
  line L96 (33.9806, -140.2615) -> (34.1848, -140.2615)
  line L97 (37.2178, -140.5603) -> (38.8614, -140.5603)
  line L98 (38.8614, -140.5603) -> (42.5967, -145.1373)
  line L99 (42.5967, -145.1373) -> (42.5967, -141.6161)
  spline S156 degree 2 poles (42.5967, -141.6161) (42.5967, -141.0534) (42.4721, -140.9139) knots 0 0 0 1 1 1
  spline S157 degree 2 poles (42.4721, -140.9139) (42.3028, -140.7247) (41.9442, -140.7247) knots 0 0 0 1 1 1
  line L100 (41.9442, -140.7247) -> (41.735, -140.7247)
  line L101 (41.735, -140.7247) -> (41.735, -140.5603)
  line L102 (41.735, -140.5603) -> (43.8517, -140.5603)
  line L103 (43.8517, -140.5603) -> (43.8517, -140.7247)
  line L104 (43.8517, -140.7247) -> (43.6376, -140.7247)
  spline S158 degree 2 poles (43.6376, -140.7247) (43.2491, -140.7247) (43.0897, -140.9587) knots 0 0 0 1 1 1
  spline S159 degree 2 poles (43.0897, -140.9587) (42.9901, -141.1032) (42.9901, -141.6161) knots 0 0 0 1 1 1
  line L105 (42.9901, -141.6161) -> (42.9901, -146.7559)
  line L106 (42.9901, -146.7559) -> (42.8307, -146.7559)
  line L107 (42.8307, -146.7559) -> (38.8116, -141.8452)
  line L108 (38.8116, -141.8452) -> (38.8116, -145.6005)
  spline S160 degree 2 poles (38.8116, -145.6005) (38.8116, -146.1632) (38.9311, -146.3027) knots 0 0 0 1 1 1
  spline S161 degree 2 poles (38.9311, -146.3027) (39.1054, -146.4919) (39.459, -146.4919) knots 0 0 0 1 1 1
  line L109 (39.459, -146.4919) -> (39.6732, -146.4919)
  line L110 (39.6732, -146.4919) -> (39.6732, -146.6563)
  line L111 (39.6732, -146.6563) -> (37.5565, -146.6563)
  line L112 (37.5565, -146.6563) -> (37.5565, -146.4919)
  line L113 (37.5565, -146.4919) -> (37.7657, -146.4919)
  spline S162 degree 2 poles (37.7657, -146.4919) (38.1591, -146.4919) (38.3185, -146.2579) knots 0 0 0 1 1 1
  spline S163 degree 2 poles (38.3185, -146.2579) (38.4181, -146.1134) (38.4181, -145.6005) knots 0 0 0 1 1 1
  line L114 (38.4181, -145.6005) -> (38.4181, -141.3621)
  spline S164 degree 2 poles (38.4181, -141.3621) (38.1541, -141.0484) (37.8802, -140.8492) (37.6113, -140.7645) knots 0 0 0 1 2 2 2
  spline S165 degree 2 poles (37.6113, -140.7645) (37.4818, -140.7247) (37.2178, -140.7247) knots 0 0 0 1 1 1
  line L115 (37.2178, -140.7247) -> (37.2178, -140.5603)
  spline S166 degree 2 poles (46.2871, -142.418) (47.2234, -142.418) (47.7862, -143.1302) knots 0 0 0 1 1 1
  spline S167 degree 2 poles (47.7862, -143.1302) (48.2693, -143.7328) (48.2693, -144.5197) knots 0 0 0 1 1 1
  spline S168 degree 2 poles (48.2693, -144.5197) (48.2693, -145.0725) (47.7364, -146.2081) (46.8101, -146.7808) (46.2373, -146.7808) knots 0 0 0 1 2 3 3 3
  spline S169 degree 2 poles (46.2373, -146.7808) (45.306, -146.7808) (44.7581, -146.0387) knots 0 0 0 1 1 1
  spline S170 degree 2 poles (44.7581, -146.0387) (44.295, -145.4162) (44.295, -144.6392) knots 0 0 0 1 1 1
  spline S171 degree 2 poles (44.295, -144.6392) (44.295, -144.0715) (44.8578, -142.9509) (45.7741, -142.418) (46.2871, -142.418) knots 0 0 0 1 2 3 3 3
  spline S172 degree 2 poles (46.1477, -142.7118) (45.9086, -142.7118) (45.4305, -142.9957) (45.1317, -143.7029) (45.1317, -144.2607) knots 0 0 0 1 2 3 3 3
  spline S173 degree 2 poles (45.1317, -144.2607) (45.1317, -145.1572) (45.8439, -146.4621) (46.4316, -146.4621) knots 0 0 0 1 2 2 2
  spline S174 degree 2 poles (46.4316, -146.4621) (46.8649, -146.4621) (47.4326, -145.7449) (47.4326, -144.8683) knots 0 0 0 1 2 2 2
  spline S175 degree 2 poles (47.4326, -144.8683) (47.4326, -143.7727) (46.9595, -143.1451) knots 0 0 0 1 1 1
  spline S176 degree 2 poles (46.9595, -143.1451) (46.6407, -142.7118) (46.1477, -142.7118) knots 0 0 0 1 1 1
  spline S177 degree 2 poles (49.883, -145.7847) (50.0921, -145.7847) (50.381, -146.0786) (50.381, -146.2828) knots 0 0 0 1 2 2 2
  spline S178 degree 2 poles (50.381, -146.2828) (50.381, -146.4919) (50.0872, -146.7808) (49.883, -146.7808) knots 0 0 0 1 2 2 2
  spline S179 degree 2 poles (49.883, -146.7808) (49.6738, -146.7808) (49.3849, -146.4919) (49.3849, -146.2828) knots 0 0 0 1 2 2 2
  spline S180 degree 2 poles (49.3849, -146.2828) (49.3849, -146.0786) (49.6738, -145.7847) (49.883, -145.7847) knots 0 0 0 1 2 2 2
  spline S181 degree 2 poles (49.8929, -142.418) (50.0971, -142.418) (50.391, -142.7118) (50.391, -142.916) knots 0 0 0 1 2 2 2
  spline S182 degree 2 poles (50.391, -142.916) (50.391, -143.1202) (50.0971, -143.4141) (49.8929, -143.4141) knots 0 0 0 1 2 2 2
  spline S183 degree 2 poles (49.8929, -143.4141) (49.6887, -143.4141) (49.3949, -143.1202) (49.3949, -142.916) knots 0 0 0 1 2 2 2
  spline S184 degree 2 poles (49.3949, -142.916) (49.3949, -142.7118) (49.6887, -142.418) (49.8929, -142.418) knots 0 0 0 1 2 2 2
  line L116 (57.6773, -144.6193) -> (55.3066, -144.6193)
  line L117 (55.3066, -144.6193) -> (54.8932, -145.5756)
  spline S185 degree 2 poles (54.8932, -145.5756) (54.7389, -145.9341) (54.7389, -146.1085) knots 0 0 0 1 1 1
  spline S186 degree 2 poles (54.7389, -146.1085) (54.7389, -146.2479) (55.0078, -146.4621) (55.4461, -146.4919) knots 0 0 0 1 2 2 2
  line L118 (55.4461, -146.4919) -> (55.4461, -146.6563)
  line L119 (55.4461, -146.6563) -> (53.5236, -146.6563)
  line L120 (53.5236, -146.6563) -> (53.5236, -146.4919)
  spline S187 degree 2 poles (53.5236, -146.4919) (53.9071, -146.4222) (54.0167, -146.3176) knots 0 0 0 1 1 1
  spline S188 degree 2 poles (54.0167, -146.3176) (54.2458, -146.0985) (54.5247, -145.4361) knots 0 0 0 1 1 1
  line L121 (54.5247, -145.4361) -> (56.6762, -140.4209)
  line L122 (56.6762, -140.4209) -> (56.8356, -140.4209)
  line L123 (56.8356, -140.4209) -> (58.9572, -145.4909)
  spline S189 degree 2 poles (58.9572, -145.4909) (59.2112, -146.1035) (59.6296, -146.467) (60.0031, -146.4919) knots 0 0 0 1 2 2 2
  line L124 (60.0031, -146.4919) -> (60.0031, -146.6563)
  line L125 (60.0031, -146.6563) -> (57.5976, -146.6563)
  line L126 (57.5976, -146.6563) -> (57.5976, -146.4919)
  spline S190 degree 2 poles (57.5976, -146.4919) (57.9612, -146.472) (58.2201, -146.2678) (58.2201, -146.1184) knots 0 0 0 1 2 2 2
  spline S191 degree 2 poles (58.2201, -146.1184) (58.2201, -145.9192) (58.0409, -145.4909) knots 0 0 0 1 1 1
  line L127 (58.0409, -145.4909) -> (57.6773, -144.6193)
  line L128 (57.5378, -144.2856) -> (56.5119, -141.8203)
  line L129 (56.5119, -141.8203) -> (55.4461, -144.2856)
  line L130 (55.4461, -144.2856) -> (57.5378, -144.2856)
  spline S192 degree 2 poles (60.4364, -143.6432) (60.4364, -142.6023) (61.064, -141.0982) (61.5869, -140.7296) knots 0 0 0 1 2 2 2
  spline S193 degree 2 poles (61.5869, -140.7296) (61.9903, -140.4358) (62.4236, -140.4358) knots 0 0 0 1 1 1
  spline S194 degree 2 poles (62.4236, -140.4358) (63.1258, -140.4358) (63.6836, -141.148) knots 0 0 0 1 1 1
  spline S195 degree 2 poles (63.6836, -141.148) (64.3809, -142.0345) (64.3809, -143.5485) knots 0 0 0 1 1 1
  spline S196 degree 2 poles (64.3809, -143.5485) (64.3809, -144.6094) (63.7683, -146.0935) (62.822, -146.7609) (62.3788, -146.7609) knots 0 0 0 1 2 3 3 3
  spline S197 degree 2 poles (62.3788, -146.7609) (61.5072, -146.7609) (60.9245, -145.7299) knots 0 0 0 1 1 1
  spline S198 degree 2 poles (60.9245, -145.7299) (60.4364, -144.8634) (60.4364, -143.6432) knots 0 0 0 1 1 1
  spline S199 degree 2 poles (61.318, -143.7577) (61.318, -145.0128) (61.6267, -145.8096) knots 0 0 0 1 1 1
  spline S200 degree 2 poles (61.6267, -145.8096) (61.8857, -146.477) (62.3937, -146.477) knots 0 0 0 1 1 1
  spline S201 degree 2 poles (62.3937, -146.477) (62.6378, -146.477) (63.1557, -146.0437) (63.2902, -145.5307) knots 0 0 0 1 2 2 2
  spline S202 degree 2 poles (63.2902, -145.5307) (63.4994, -144.7588) (63.4994, -143.3543) knots 0 0 0 1 1 1
  spline S203 degree 2 poles (63.4994, -143.3543) (63.4994, -142.3084) (63.2852, -141.6161) knots 0 0 0 1 1 1
  spline S204 degree 2 poles (63.2852, -141.6161) (63.1209, -141.0982) (62.8669, -140.884) knots 0 0 0 1 1 1
  spline S205 degree 2 poles (62.8669, -140.884) (62.6826, -140.7346) (62.4186, -140.7346) knots 0 0 0 1 1 1
  spline S206 degree 2 poles (62.4186, -140.7346) (62.1148, -140.7346) (61.8758, -141.0085) knots 0 0 0 1 1 1
  spline S207 degree 2 poles (61.8758, -141.0085) (61.552, -141.3821) (61.318, -142.9808) (61.318, -143.7577) knots 0 0 0 1 2 2 2
  line L131 (68.7089, -140.5603) -> (68.3602, -141.3223)
  line L132 (68.3602, -141.3223) -> (66.5274, -141.3223)
  line L133 (66.5274, -141.3223) -> (66.124, -142.1391)
  spline S208 degree 2 poles (66.124, -142.1391) (67.3143, -142.3134) (68.0116, -143.0256) knots 0 0 0 1 1 1
  spline S209 degree 2 poles (68.0116, -143.0256) (68.6092, -143.6382) (68.6092, -144.4649) knots 0 0 0 1 1 1
  spline S210 degree 2 poles (68.6092, -144.4649) (68.6092, -144.943) (68.2158, -145.7648) (67.6231, -146.3376) (67.2596, -146.5119) knots 0 0 0 1 2 3 3 3
  spline S211 degree 2 poles (67.2596, -146.5119) (66.7416, -146.7609) (66.1987, -146.7609) knots 0 0 0 1 1 1
  spline S212 degree 2 poles (66.1987, -146.7609) (65.6459, -146.7609) (65.1479, -146.3874) (65.1479, -146.1632) knots 0 0 0 1 2 2 2
  spline S213 degree 2 poles (65.1479, -146.1632) (65.1479, -146.0387) (65.3521, -145.8445) (65.5114, -145.8445) knots 0 0 0 1 2 2 2
  spline S214 degree 2 poles (65.5114, -145.8445) (65.626, -145.8445) (65.8053, -145.9192) (66.0145, -146.0686) knots 0 0 0 1 2 2 2
  spline S215 degree 2 poles (66.0145, -146.0686) (66.3531, -146.2977) (66.7018, -146.3027) knots 0 0 0 1 1 1
  spline S216 degree 2 poles (66.7018, -146.3027) (67.2247, -146.3027) (68.0265, -145.5058) (68.0265, -144.9331) knots 0 0 0 1 2 2 2
  spline S217 degree 2 poles (68.0265, -144.9331) (68.0265, -144.3803) (67.3143, -143.419) (66.6868, -143.1601) knots 0 0 0 1 2 2 2
  spline S218 degree 2 poles (66.6868, -143.1601) (66.1987, -142.9559) (65.3521, -142.926) knots 0 0 0 1 1 1
  line L134 (65.3521, -142.926) -> (66.5225, -140.5603)
  line L135 (66.5225, -140.5603) -> (68.7089, -140.5603)
  spline S219 degree 2 poles (69.6501, -143.6432) (69.6501, -142.6023) (70.2777, -141.0982) (70.8006, -140.7296) knots 0 0 0 1 2 2 2
  spline S220 degree 2 poles (70.8006, -140.7296) (71.204, -140.4358) (71.6373, -140.4358) knots 0 0 0 1 1 1
  spline S221 degree 2 poles (71.6373, -140.4358) (72.3396, -140.4358) (72.8974, -141.148) knots 0 0 0 1 1 1
  spline S222 degree 2 poles (72.8974, -141.148) (73.5946, -142.0345) (73.5946, -143.5485) knots 0 0 0 1 1 1
  spline S223 degree 2 poles (73.5946, -143.5485) (73.5946, -144.6094) (72.982, -146.0935) (72.0358, -146.7609) (71.5925, -146.7609) knots 0 0 0 1 2 3 3 3
  spline S224 degree 2 poles (71.5925, -146.7609) (70.7209, -146.7609) (70.1382, -145.7299) knots 0 0 0 1 1 1
  spline S225 degree 2 poles (70.1382, -145.7299) (69.6501, -144.8634) (69.6501, -143.6432) knots 0 0 0 1 1 1
  spline S226 degree 2 poles (70.5317, -143.7577) (70.5317, -145.0128) (70.8405, -145.8096) knots 0 0 0 1 1 1
  spline S227 degree 2 poles (70.8405, -145.8096) (71.0994, -146.477) (71.6074, -146.477) knots 0 0 0 1 1 1
  spline S228 degree 2 poles (71.6074, -146.477) (71.8515, -146.477) (72.3694, -146.0437) (72.5039, -145.5307) knots 0 0 0 1 2 2 2
  spline S229 degree 2 poles (72.5039, -145.5307) (72.7131, -144.7588) (72.7131, -143.3543) knots 0 0 0 1 1 1
  spline S230 degree 2 poles (72.7131, -143.3543) (72.7131, -142.3084) (72.4989, -141.6161) knots 0 0 0 1 1 1
  spline S231 degree 2 poles (72.4989, -141.6161) (72.3346, -141.0982) (72.0806, -140.884) knots 0 0 0 1 1 1
  spline S232 degree 2 poles (72.0806, -140.884) (71.8963, -140.7346) (71.6323, -140.7346) knots 0 0 0 1 1 1
  spline S233 degree 2 poles (71.6323, -140.7346) (71.3285, -140.7346) (71.0895, -141.0085) knots 0 0 0 1 1 1
  spline S234 degree 2 poles (71.0895, -141.0085) (70.7658, -141.3821) (70.5317, -142.9808) (70.5317, -143.7577) knots 0 0 0 1 2 2 2
  spline S235 degree 2 poles (74.257, -143.6432) (74.257, -142.6023) (74.8845, -141.0982) (75.4075, -140.7296) knots 0 0 0 1 2 2 2
  spline S236 degree 2 poles (75.4075, -140.7296) (75.8109, -140.4358) (76.2442, -140.4358) knots 0 0 0 1 1 1
  spline S237 degree 2 poles (76.2442, -140.4358) (76.9464, -140.4358) (77.5042, -141.148) knots 0 0 0 1 1 1
  spline S238 degree 2 poles (77.5042, -141.148) (78.2015, -142.0345) (78.2015, -143.5485) knots 0 0 0 1 1 1
  spline S239 degree 2 poles (78.2015, -143.5485) (78.2015, -144.6094) (77.5889, -146.0935) (76.6426, -146.7609) (76.1994, -146.7609) knots 0 0 0 1 2 3 3 3
  spline S240 degree 2 poles (76.1994, -146.7609) (75.3278, -146.7609) (74.7451, -145.7299) knots 0 0 0 1 1 1
  spline S241 degree 2 poles (74.7451, -145.7299) (74.257, -144.8634) (74.257, -143.6432) knots 0 0 0 1 1 1
  spline S242 degree 2 poles (75.1385, -143.7577) (75.1385, -145.0128) (75.4473, -145.8096) knots 0 0 0 1 1 1
  spline S243 degree 2 poles (75.4473, -145.8096) (75.7063, -146.477) (76.2143, -146.477) knots 0 0 0 1 1 1
  spline S244 degree 2 poles (76.2143, -146.477) (76.4583, -146.477) (76.9763, -146.0437) (77.1108, -145.5307) knots 0 0 0 1 2 2 2
  spline S245 degree 2 poles (77.1108, -145.5307) (77.32, -144.7588) (77.32, -143.3543) knots 0 0 0 1 1 1
  spline S246 degree 2 poles (77.32, -143.3543) (77.32, -142.3084) (77.1058, -141.6161) knots 0 0 0 1 1 1
  spline S247 degree 2 poles (77.1058, -141.6161) (76.9414, -141.0982) (76.6874, -140.884) knots 0 0 0 1 1 1
  spline S248 degree 2 poles (76.6874, -140.884) (76.5032, -140.7346) (76.2392, -140.7346) knots 0 0 0 1 1 1
  spline S249 degree 2 poles (76.2392, -140.7346) (75.9354, -140.7346) (75.6963, -141.0085) knots 0 0 0 1 1 1
  spline S250 degree 2 poles (75.6963, -141.0085) (75.3726, -141.3821) (75.1385, -142.9808) (75.1385, -143.7577) knots 0 0 0 1 2 2 2
  spline S251 degree 2 poles (78.8639, -143.6432) (78.8639, -142.6023) (79.4914, -141.0982) (80.0143, -140.7296) knots 0 0 0 1 2 2 2
  spline S252 degree 2 poles (80.0143, -140.7296) (80.4178, -140.4358) (80.8511, -140.4358) knots 0 0 0 1 1 1
  spline S253 degree 2 poles (80.8511, -140.4358) (81.5533, -140.4358) (82.1111, -141.148) knots 0 0 0 1 1 1
  spline S254 degree 2 poles (82.1111, -141.148) (82.8083, -142.0345) (82.8083, -143.5485) knots 0 0 0 1 1 1
  spline S255 degree 2 poles (82.8083, -143.5485) (82.8083, -144.6094) (82.1958, -146.0935) (81.2495, -146.7609) (80.8062, -146.7609) knots 0 0 0 1 2 3 3 3
  spline S256 degree 2 poles (80.8062, -146.7609) (79.9347, -146.7609) (79.352, -145.7299) knots 0 0 0 1 1 1
  spline S257 degree 2 poles (79.352, -145.7299) (78.8639, -144.8634) (78.8639, -143.6432) knots 0 0 0 1 1 1
  spline S258 degree 2 poles (79.7454, -143.7577) (79.7454, -145.0128) (80.0542, -145.8096) knots 0 0 0 1 1 1
  spline S259 degree 2 poles (80.0542, -145.8096) (80.3132, -146.477) (80.8212, -146.477) knots 0 0 0 1 1 1
  spline S260 degree 2 poles (80.8212, -146.477) (81.0652, -146.477) (81.5832, -146.0437) (81.7176, -145.5307) knots 0 0 0 1 2 2 2
  spline S261 degree 2 poles (81.7176, -145.5307) (81.9268, -144.7588) (81.9268, -143.3543) knots 0 0 0 1 1 1
  spline S262 degree 2 poles (81.9268, -143.3543) (81.9268, -142.3084) (81.7127, -141.6161) knots 0 0 0 1 1 1
  spline S263 degree 2 poles (81.7127, -141.6161) (81.5483, -141.0982) (81.2943, -140.884) knots 0 0 0 1 1 1
  spline S264 degree 2 poles (81.2943, -140.884) (81.11, -140.7346) (80.8461, -140.7346) knots 0 0 0 1 1 1
  spline S265 degree 2 poles (80.8461, -140.7346) (80.5423, -140.7346) (80.3032, -141.0085) knots 0 0 0 1 1 1
  spline S266 degree 2 poles (80.3032, -141.0085) (79.9795, -141.3821) (79.7454, -142.9808) (79.7454, -143.7577) knots 0 0 0 1 2 2 2
  spline S267 degree 2 poles (83.4707, -143.6432) (83.4707, -142.6023) (84.0983, -141.0982) (84.6212, -140.7296) knots 0 0 0 1 2 2 2
  spline S268 degree 2 poles (84.6212, -140.7296) (85.0246, -140.4358) (85.4579, -140.4358) knots 0 0 0 1 1 1
  spline S269 degree 2 poles (85.4579, -140.4358) (86.1601, -140.4358) (86.718, -141.148) knots 0 0 0 1 1 1
  spline S270 degree 2 poles (86.718, -141.148) (87.4152, -142.0345) (87.4152, -143.5485) knots 0 0 0 1 1 1
  spline S271 degree 2 poles (87.4152, -143.5485) (87.4152, -144.6094) (86.8026, -146.0935) (85.8563, -146.7609) (85.4131, -146.7609) knots 0 0 0 1 2 3 3 3
  spline S272 degree 2 poles (85.4131, -146.7609) (84.5415, -146.7609) (83.9588, -145.7299) knots 0 0 0 1 1 1
  spline S273 degree 2 poles (83.9588, -145.7299) (83.4707, -144.8634) (83.4707, -143.6432) knots 0 0 0 1 1 1
  spline S274 degree 2 poles (84.3523, -143.7577) (84.3523, -145.0128) (84.6611, -145.8096) knots 0 0 0 1 1 1
  spline S275 degree 2 poles (84.6611, -145.8096) (84.92, -146.477) (85.428, -146.477) knots 0 0 0 1 1 1
  spline S276 degree 2 poles (85.428, -146.477) (85.6721, -146.477) (86.19, -146.0437) (86.3245, -145.5307) knots 0 0 0 1 2 2 2
  spline S277 degree 2 poles (86.3245, -145.5307) (86.5337, -144.7588) (86.5337, -143.3543) knots 0 0 0 1 1 1
  spline S278 degree 2 poles (86.5337, -143.3543) (86.5337, -142.3084) (86.3195, -141.6161) knots 0 0 0 1 1 1
  spline S279 degree 2 poles (86.3195, -141.6161) (86.1552, -141.0982) (85.9012, -140.884) knots 0 0 0 1 1 1
  spline S280 degree 2 poles (85.9012, -140.884) (85.7169, -140.7346) (85.4529, -140.7346) knots 0 0 0 1 1 1
  spline S281 degree 2 poles (85.4529, -140.7346) (85.1491, -140.7346) (84.9101, -141.0085) knots 0 0 0 1 1 1
  spline S282 degree 2 poles (84.9101, -141.0085) (84.5863, -141.3821) (84.3523, -142.9808) (84.3523, -143.7577) knots 0 0 0 1 2 2 2
  line L136 (91.9673, -145.4859) -> (91.539, -146.6563)
  line L137 (91.539, -146.6563) -> (87.9431, -146.6563)
  line L138 (87.9431, -146.6563) -> (87.9431, -146.4919)
  spline S283 degree 2 poles (87.9431, -146.4919) (89.5319, -145.0427) (90.8268, -143.2099) (90.8268, -142.4479) knots 0 0 0 1 2 2 2
  spline S284 degree 2 poles (90.8268, -142.4479) (90.8268, -141.8701) (90.1146, -141.1231) (89.6215, -141.1231) knots 0 0 0 1 2 2 2
  spline S285 degree 2 poles (89.6215, -141.1231) (89.1683, -141.1231) (88.4561, -141.651) (88.2818, -142.159) knots 0 0 0 1 2 2 2
  line L139 (88.2818, -142.159) -> (88.1174, -142.159)
  spline S286 degree 2 poles (88.1174, -142.159) (88.232, -141.3273) (89.1583, -140.4358) (89.8556, -140.4358) knots 0 0 0 1 2 2 2
  spline S287 degree 2 poles (89.8556, -140.4358) (90.5977, -140.4358) (91.5938, -141.387) (91.5938, -142.0345) knots 0 0 0 1 2 2 2
  spline S288 degree 2 poles (91.5938, -142.0345) (91.5938, -142.4977) (91.3796, -142.9609) knots 0 0 0 1 1 1
  spline S289 degree 2 poles (91.3796, -142.9609) (91.0459, -143.688) (90.2989, -144.5048) knots 0 0 0 1 1 1
  spline S290 degree 2 poles (90.2989, -144.5048) (89.1783, -145.725) (88.8994, -145.979) knots 0 0 0 1 1 1
  line L140 (88.8994, -145.979) -> (90.4931, -145.979)
  spline S291 degree 2 poles (90.4931, -145.979) (90.9812, -145.979) (91.3696, -145.9092) (91.6834, -145.6851) (91.8029, -145.4859) knots 0 0 0 1 2 3 3 3
  line L141 (91.8029, -145.4859) -> (91.9673, -145.4859)
  line L142 (29.5381, -154.261) -> (27.1674, -154.261)
  line L143 (27.1674, -154.261) -> (26.754, -155.2172)
  spline S292 degree 2 poles (26.754, -155.2172) (26.5996, -155.5758) (26.5996, -155.7502) knots 0 0 0 1 1 1